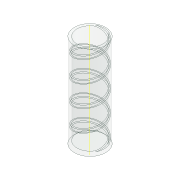
# Autodesk Inventor part: Screw
Saved by Autodesk Inventor 2020.4 (Build 244396000, 396)
## iProperties
Created: 2022-05-29
Part Number: Screw
Material: Generic
Document SubType Name: Modeling
Designer: david
Density: 1 g/cm^3
Appearance: Clear
Author: david
Autodesk Inventor part; units mm, degrees
ref_plane "YZ Plane" through (0, 0, 0) normal (1, 0, 0) x (0, 1, 0)
ref_plane "XZ Plane" through (0, 0, 0) normal (0, 1, 0) x (-1, 0, 0)
ref_plane "XY Plane" through (0, 0, 0) normal (0, 0, 1) x (1, 0, 0)
sketch "Sketch1" plane through (0, 0, 0) normal (0, 1, 0) x (-1, 0, 0)
  circle A0 centre (0, 0) radius 15.5575
  circle A1 centre (0, 0) radius 18.7325
  line L0 (0, 0) -> (0, -6.8592)
  line L1 (7.62, -17.1126) -> (7.62, 17.1126)
  line L2 (-7.62, -17.1126) -> (-7.62, 17.1126)
  circle A2 centre (0, 0) radius 17.145
  dimension "d0" = 31.115
  dimension "d1" = 3.175
  dimension "d2" = 7.62
  dimension "d3" = 1.5875
  constraints: 6 end point, 3 centre point, 3 coincident, 2 point on circle, 2 symmetric about line, 2 vertical
  measures "d0" diameter of A0
  measures "d1" radial gap between concentric circles of A1 A0
  measures "d2" distance between parallel lines of L0 L1
  measures "d3" radial gap between concentric circles of A2 A0
extrude "Extrusion1" add sketch "Sketch1" along normal blind 3.175 contours A0 L1 | L1 A0 L2 | L2 A0
extrude "Extrusion2" add sketch "Sketch1" along normal blind 111.125 contours A0 L1 A2 | A0 L2 A2 L1 | L1 A2 L2 A0 | A0 L2 A2 | A2 L2 A1 L1 | L1 A1 A2 | L1 A1 L2 A2 | A2 L2 A1
sketch "Sketch2" plane through (0, 111.125, 0) normal (0, 1, 0) x (1, 0, 0)
  circle A0 centre (0, 0) radius 18.7325 projected
  circle A1 centre (0, 0) radius 15.5575 projected
  circle A2 centre (0, 0) radius 18.7325 projected
  circle A3 centre (0, 0) radius 15.5575 projected
  circle A4 centre (0, 0) radius 15.5575 projected
  arc A5 (7.62, 13.5636) -> (-7.62, 13.5636) centre (0, 0) ccw
  arc A6 (7.62, 15.3586) -> (-7.62, 15.3586) centre (0, 0) ccw
  line L0 (-7.62, 13.5636) -> (-7.62, 15.3586)
  line L1 (7.62, 15.3586) -> (7.62, 13.5636)
  constraints: 6 point on circle, 4 end point, 2 centre point, 2 coincident
coil "Coil1" sketch "Sketch2" operation cut axis through (0, -10, 0) along (0, -1, 0) pitch 25.4 turns 4.25 hand right contours A1 L0 A6 L1
body "Solid1"
